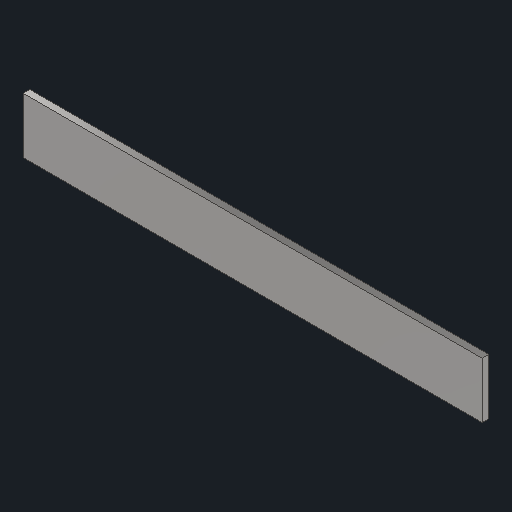
# Autodesk Inventor part: FrameBottomBeam
Saved by Autodesk Inventor 2024 (Build 280153000, 153)
## iProperties
Created: 2025-02-07
Part Number: FrameBottomBeam
Material: Stainless Steel
Document SubType Name: Sheet Metal
Designer: Tommy Rohmann
Density: 8 g/cm^3
Appearance: Semi-Polished
Sheet Metal Rule: Default
Author: Tommy Rohmann
Autodesk Inventor part; units mm, degrees
ref_plane "YZ Plane" through (0, 0, 0) normal (1, 0, 0) x (0, 1, 0)
ref_plane "XZ Plane" through (0, 0, 0) normal (0, 1, 0) x (-1, 0, 0)
ref_plane "XY Plane" through (0, 0, 0) normal (0, 0, 1) x (1, 0, 0)
sketch "FrameBottomBeam" plane through (0, 0, 0) normal (0, 0, 1) x (1, 0, 0)
  line L0 (104.1884, 9.7512) -> (104.1884, -15.6488)
  line L1 (-0.5866, -15.6488) -> (-0.5866, 9.7512)
  line L2 (104.1884, 9.7512) -> (-0.5866, 9.7512)
  line L3 (104.1884, -15.6488) -> (-0.5866, -15.6488)
  line L4 (73.9116, -15.6488) -> (73.9116, 9.7512)
  line L5 (-105.3616, 9.7512) -> (-105.3616, -15.6488)
  line L6 (-105.3616, 9.7512) -> (-0.5866, 9.7512)
  line L7 (-105.3616, -15.6488) -> (-0.5866, -15.6488)
  line L8 (-75.0848, -15.6488) -> (-75.0848, 9.7512)
  point P0 (-8.6642, 25.0995)
  dimension "d227" = 209.55
  dimension "d228" = 148.9964
  dimension "d244" = 25.4
  measures "d227" diameter of L0 L1
  measures "d228" diameter of L4 L1
  measures "d244" distance between parallel lines of L3 L2
derived "LAYOUT.ipt"
sketch "Sketch1" plane through (0, 0, 0) normal (0, 0, 1) x (1, 0, 0)
  line L0 (104.1884, 9.7512) -> (104.1884, -15.6488)
  line L1 (-0.5866, -15.6488) -> (-0.5866, 9.7512)
  line L2 (104.1884, 9.7512) -> (-0.5866, 9.7512)
  line L3 (104.1884, -15.6488) -> (-0.5866, -15.6488)
  line L4 (73.9116, -15.6488) -> (73.9116, 9.7512)
  line L5 (-105.3616, 9.7512) -> (-105.3616, -15.6488)
  line L6 (-105.3616, 9.7512) -> (-0.5866, 9.7512)
  line L7 (-105.3616, -15.6488) -> (-0.5866, -15.6488)
  line L8 (-75.0848, -15.6488) -> (-75.0848, 9.7512)
extrude "Plate1" add sketch "Sketch1" along normal blind 3.048
equation "\"d3\" = Thickness"
equation "\"BendRadius\" = Thickness"
equation "\"BendReliefWidth\" = Thickness"
equation "\"BendReliefDepth\" = 0.5 * Thickness"
equation "\"CornerReliefSize\" = 4 * Thickness"
equation "\"MinimumRemnant\" = 2 * Thickness"
equation "\"TransitionRadius\" = BendRadius"
equation "\"JacobiRadiusSize\" = BendRadius"
equation "\"GapSize\" = Thickness"
equation "\"Thickness\" = 3.048"
body "Solid2"
